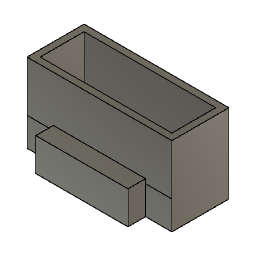
Diaper Station Wheel holders v4 (Autodesk Fusion 360 design; units mm, degrees)
Autodesk Fusion 360 part; units mm, degrees
sketch "Sketch1" plane through (0, 0, 0) normal (0, 0, 1) x (1, 0, 0)
  line L0 (9.2775, 41.8926) -> (69.2775, 41.8926)
  line L1 (69.2775, 41.8926) -> (69.2775, 21.8926)
  line L2 (69.2775, 21.8926) -> (9.2775, 21.8926)
  line L3 (9.2775, 21.8926) -> (9.2775, 41.8926)
  line L4 (72.2775, 18.8926) -> (6.2775, 18.8926)
  line L5 (6.2775, 18.8926) -> (6.2775, 44.8926)
  line L6 (6.2775, 44.8926) -> (72.2775, 44.8926)
  line L7 (72.2775, 44.8926) -> (72.2775, 18.8926)
  line L8 (18.2775, 52.8926) -> (60.2775, 52.8926)
  line L9 (60.2775, 52.8926) -> (60.2775, 10.8926)
  line L10 (60.2775, 10.8926) -> (18.2775, 10.8926)
  line L11 (18.2775, 10.8926) -> (18.2775, 52.8926)
  line L12 (39.2775, 41.8926) -> (39.2775, 21.8926) construction
  line L13 (9.2775, 31.8926) -> (69.2775, 31.8926) construction
  line L14 (18.2775, 31.8926) -> (60.2775, 31.8926) construction
  line L15 (39.2775, 10.8926) -> (39.2775, 52.8926) construction
  point P0 (39.2775, 31.8926)
  point P1 (39.2775, 31.8926)
  dimension "d1" = 60
  dimension "d2" = 20
  dimension "d3" = -3
  dimension "d4" = 42
  dimension "d5" = 42
  constraint horizontal L0
  constraint vertical L1
  constraint horizontal L2
  constraint vertical L3
  constraint horizontal L8
  constraint vertical L9
  constraint horizontal L10
  constraint vertical L11
  constraint midpoint L0 L12.start
  constraint midpoint L2 L12.end
  constraint midpoint L3 L13.start
  constraint midpoint L1 L13.end
  constraint midpoint L13 P1
  constraint midpoint L11 L14.start
  constraint midpoint L9 L14.end
  constraint midpoint L10 L15.start
  constraint midpoint L8 L15.end
  constraint midpoint L14 P1
  measures "d1" distance of L0.start L0.end
  measures "d2" distance of L0.start L2.end
  measures "d4" distance of L9 L11
  measures "d5" distance of L8 L10
extrude "Extrude1" add sketch "Sketch1" along normal blind 3 contours L0 L2 L3 L11 | L0 L2 L9 L11 | L0 L1 L2 L9 makes body 1
extrude "Extrude2" add sketch "Sketch1" along normal blind 10 contours L0 L2 L3 L4 L5 L6 L11 | L0 L6 L9 L11 | L0 L1 L2 L4 L6 L7 L9 | L2 L4 L9 L11 bodies 1
extrude "Extrude3" add sketch "Sketch1" against normal blind 3 separate body contours L0 L6 L9 L11 | L0 L2 L9 L11 | L2 L4 L9 L11 | L6 L8 L9 L11 | L4 L9 L10 L11 makes body 2
extrude "Extrude4" add sketch "Sketch1" against normal blind 3 contours L0 L2 L3 L4 L5 L6 L11 | L0 L2 L3 L11 | L0 L1 L2 L4 L6 L7 L9 | L0 L1 L2 L9 bodies 1 2
hole "Hole1" at (54.7775, 16.3926, 0) direction (0, 0, -1) diameter 4.5 depth 10 tip angle 118 bodies 1
hole "Hole4" at (23.7775, 16.3926, -3) direction (0, 0, 1) diameter 5 depth 5 tip angle 118 bodies 1
extrude "Extrude5" add 1 faces at (34.3565, 11.9297, 0) along direction (0, 0, 1) blind 10 on bodies 1 bodies 1
delete_face "DeleteFace1" 1 faces at (23.9021, 18.8895, 5.6667) on bodies 1
hole "Hole5" at (23.7775, 16.3926, -3) direction (0, 0, 1) diameter 5 depth 10 tip angle 118 bodies 1
delete_face "DeleteFace2" 1 faces at (54.8897, 14.1454, 5.6667) on bodies 1
hole "Hole6" at (54.7775, 16.3926, -3) direction (0, 0, 1) diameter 5 depth 10 tip angle 118 bodies 1
ref_plane "WorkPlane1" through (12.2775, 18.8926, 3.5) normal (0, -1, 0) x (1, 0, 0)
split_face "SplitFace1" 1 faces at (32.2775, 16.226, 10) by plane through (12.2775, 18.8926, 3.5) normal (0, -1, 0) on bodies 1
extrude "Extrude6" add 1 faces at (32.2775, 20.8926, 10) along direction (0, 0, 1) blind 23 on bodies 1 bodies 1
extrude "Extrude7" add 1 faces at (32.2775, 16.226, 10) along direction (0, 0, 1) blind 2 on bodies 1 bodies 1
extrude "Extrude8" add 1 faces at (46.2775, 50.226, 0) along direction (0, 0, 1) blind 12 on bodies 1 bodies 1
ref_plane "WorkPlane2" through (39.2775, 31.8926, 4.5) normal (0, -1, 0) x (-1, 0, 0)
mirror "Mirror1" about plane through (39.2775, 31.8926, 4.5) normal (0, -1, 0) of "Hole5", "Hole6"
